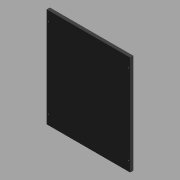
# Autodesk Inventor part: box_back
Saved by Autodesk Inventor 2019 (Build 230136000, 136)
## iProperties
Part Number: box_back
Material: Generic
Document SubType Name: Modeling
Designer: Javi
Appearance: Default
Author: Javi
Autodesk Inventor part; units mm, degrees
ref_plane "YZ Plane" through (0, 0, 0) normal (1, 0, 0) x (0, 1, 0)
ref_plane "XZ Plane" through (0, 0, 0) normal (0, 1, 0) x (-1, 0, 0)
ref_plane "XY Plane" through (0, 0, 0) normal (0, 0, 1) x (1, 0, 0)
sketch "Sketch1" plane through (0, 0, 0) normal (1, 0, 0) x (0, 1, 0)
  line L0 (0, 0) -> (310, 0)
  line L1 (310, 0) -> (310, -10)
  line L2 (310, -10) -> (0, -10)
  line L3 (0, -10) -> (0, 0)
  dimension "d0" = 310
  dimension "d1" = 10
  constraints: 8 end point, 2 parallel, 1 horizontal, 1 perpendicular
  measures "d0" distance of L1.end L2.end
  measures "d1" distance of L0.end L1.end
extrude "Extrusion1" add sketch "Sketch1" along normal blind 260
sketch "Sketch2" plane through (0, 0, -10) normal (0, 0, -1) x (-1, 0, 0)
  circle A0 centre (-255, 280) radius 2
  line L0 (-260, 0) -> (-260, 310) projected
  line L1 (0, 310) -> (-260, 310) projected
  circle A1 centre (-255, 30) radius 2
  circle A2 centre (-5, 280) radius 2
  circle A3 centre (-5, 30) radius 2
  point P0 (0, 0)
  dimension "d4" = 4
  dimension "d5" = 5
  dimension "d6" = 30
  dimension "d9" = 250
  dimension "d12" = 250
  constraints: 4 centre point, 1 horizontal, 1 vertical, 6 other
  measures "d4" diameter of A0
  measures "d5" distance from line of L0 A0.centre
  measures "d6" distance from line of L1 A0.centre
  measures "d9" distance of A0.centre A1.centre
  measures "d12" distance of A0.centre A2.centre
extrude "Extrusion2" cut sketch "Sketch2" against normal through all
sketch "Sketch3" plane through (0, 0, -10) normal (0, -1, 0) x (1, 0, 0)
  circle A0 centre (30, 5) radius 2
  line L0 (0, 0) -> (260, 0) projected
  line L1 (0, 0) -> (0, 10) projected
  circle A1 centre (230, 5) radius 2
  dimension "d17" = 4
  dimension "d18" = 5
  dimension "d19" = 30
  dimension "d22" = 200
  constraints: 2 centre point, 1 horizontal, 2 other
  measures "d17" diameter of A0
  measures "d18" distance from line of L0 A0.centre
  measures "d19" distance from line of L1 A0.centre
  measures "d22" distance of A0.centre A1.centre
extrude "Extrusion3" cut sketch "Sketch3" against normal blind 20
body "Solid1"
